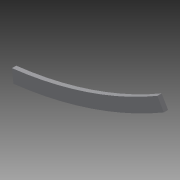
# Autodesk Inventor part: nd-12
Saved by Autodesk Inventor 2015 (Build 190159000, 159)
## iProperties
Created: 2014-07-02
Part Number: nd-12
Material: Generic
Document SubType Name: Modeling
Designer: peter
Density: 1 g/cm^3
Appearance: Default
Author: peter
Autodesk Inventor part; units mm, degrees
ref_plane "YZ Plane" through (0, 0, 0) normal (1, 0, 0) x (0, 1, 0)
ref_plane "XZ Plane" through (0, 0, 0) normal (0, 1, 0) x (-1, 0, 0)
ref_plane "XY Plane" through (0, 0, 0) normal (0, 0, 1) x (1, 0, 0)
sketch "Sketch1" plane through (0, 0, 0) normal (0, 0, 1) x (1, 0, 0)
  arc A0 (0.0856, 56.7095) -> (645.7753, 272.8727) centre (-196.1119, 1715.1948) ccw
  line L0 (0.0856, 56.7095) -> (6.7993, -0.0427)
  arc A1 (6.7993, -0.0427) -> (674.5197, 223.4775) centre (-196.091, 1715.1488) ccw
  line L1 (674.5197, 223.4775) -> (645.7753, 272.8727)
  point P0 (0, 0)
  constraints: 4 end point, 4 point on circle, 2 centre point
extrude "Extrusion1" add sketch "Sketch1" along normal blind 19.05
body "Solid1"
